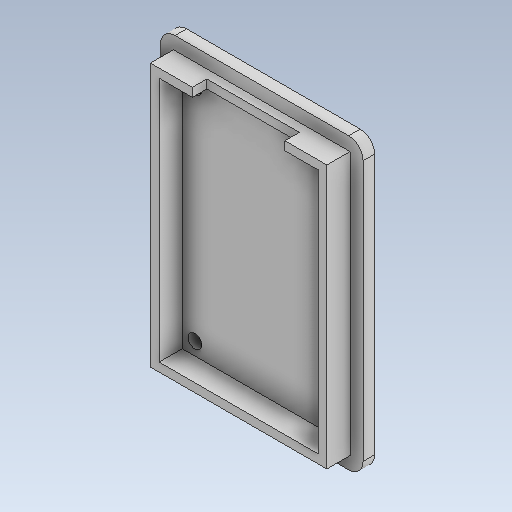
# Autodesk Inventor part: EnclosureTop
Saved by Autodesk Inventor 2020 (Build 240168000, 168)
## iProperties
Created: 2019-09-23
Part Number: EnclosureTop
Material: Generic
Document SubType Name: Modeling
Designer: veloxstatera
Density: 1 g/cm^3
Appearance: Default
Author: veloxstatera
Autodesk Inventor part; units mm, degrees
ref_plane "YZ Plane" through (0, 0, 0) normal (1, 0, 0) x (0, 1, 0)
ref_plane "XZ Plane" through (0, 0, 0) normal (0, 1, 0) x (-1, 0, 0)
ref_plane "XY Plane" through (0, 0, 0) normal (0, 0, 1) x (1, 0, 0)
sketch "Sketch1" plane through (0, 0, 0) normal (0, 0, 1) x (1, 0, 0)
  line L0 (-44.45, 63.5) -> (44.45, 63.5)
  line L1 (44.45, 63.5) -> (44.45, -63.5)
  line L2 (44.45, -63.5) -> (-44.45, -63.5)
  line L3 (-44.45, -63.5) -> (-44.45, 63.5)
  line L4 (0, 63.5) -> (0, -63.5) construction
  point P0 (0, 0)
  point P1 (0, 0)
  dimension "d0" = 88.9
  dimension "d1" = 127
  constraints: 10 end point, 3 midpoint, 2 parallel, 1 coincident, 1 horizontal, 1 perpendicular
  measures "d0" distance of L0.start L0.end
  measures "d1" distance of L0.end L1.end
extrude "Extrusion1" add sketch "Sketch1" along normal blind 5.08
fillet "Fillet1" radius 6.35 4 edges at (44.45, 63.5, 2.54) (-44.45, 63.5, 2.54) (44.45, -63.5, 2.54) (-44.45, -63.5, 2.54)
sketch "Sketch2" plane through (0, 0, 5.08) normal (0, 0, 1) x (1, 0, 0)
  line L0 (-38.735, 57.785) -> (38.735, 57.785)
  line L1 (38.735, 57.785) -> (38.735, -57.785)
  line L2 (38.735, -57.785) -> (-38.735, -57.785)
  line L3 (-38.735, -57.785) -> (-38.735, 57.785)
  line L4 (38.1, 63.5) -> (-38.1, 63.5) construction
  line L5 (44.45, -57.15) -> (44.45, 57.15) construction
  line L6 (0, 57.785) -> (0, -57.785) construction
  point P0 (0, 0)
  point P1 (0, 0)
  dimension "d5" = 77.47
  dimension "d6" = 115.57
  constraints: 10 end point, 3 midpoint, 2 parallel, 1 coincident, 1 horizontal, 1 perpendicular
  measures "d5" distance of L0.start L0.end
  measures "d6" distance of L0.end L1.end
extrude "Extrusion2" add sketch "Sketch2" along normal blind 10.16
sketch "Sketch3" plane through (0, 0, 15.24) normal (0, 0, 1) x (1, 0, 0)
  line L0 (-34.925, 53.975) -> (34.925, 53.975)
  line L1 (34.925, 53.975) -> (34.925, -53.975)
  line L2 (34.925, -53.975) -> (-34.925, -53.975)
  line L3 (-34.925, -53.975) -> (-34.925, 53.975)
  line L4 (0, -53.975) -> (0, 53.975) construction
  line L5 (38.735, 57.785) -> (-38.735, 57.785) projected
  line L6 (-38.735, 57.785) -> (-38.735, -57.785) projected
  point P0 (0, 0)
  point P1 (0, 0)
  dimension "d9" = 3.81
  dimension "d10" = 3.81
  constraints: 10 end point, 3 midpoint, 2 parallel, 1 coincident, 1 horizontal, 1 perpendicular
  measures "d9" distance between parallel lines of L5 L0
  measures "d10" distance between parallel lines of L6 L3
extrude "Extrusion3" cut sketch "Sketch3" against normal blind 10.16
sketch "Sketch4" plane through (-38.735, 57.785, 5.08) normal (0, 1, 0) x (1, 0, 0)
  line L0 (77.47, -10.16) -> (0, -10.16) projected
  line L1 (59.055, -10.16) -> (18.415, -10.16)
  line L2 (18.415, -10.16) -> (18.415, -3.81)
  line L3 (18.415, -3.81) -> (59.055, -3.81)
  line L4 (59.055, -3.81) -> (59.055, -10.16)
  point P0 (38.735, 5.08)
  point P1 (38.735, -10.16)
  dimension "d13" = 40.64
  dimension "d14" = 6.35
  constraints: 8 end point, 2 midpoint, 2 parallel, 1 horizontal, 1 perpendicular, 1 point on line
  measures "d13" distance of L2.end L3.end
  measures "d14" distance of L3.end L1.start
extrude "Extrusion4" cut sketch "Sketch4" against normal blind 10.16
sketch "Sketch5" plane through (0, 0, 5.08) normal (0, 0, 1) x (1, 0, 0)
  circle A0 centre (-29.325, 48.375) radius 3
  line L0 (20.32, 53.975) -> (-20.32, 53.975) construction
  line L1 (0, 53.975) -> (0, 7.6098) construction
  line L2 (0, 0) -> (12.3821, 0) construction
  line L3 (-34.925, 53.975) -> (-20.32, 53.975) construction
  line L4 (-34.925, -53.975) -> (-34.925, 53.975) construction
  circle A1 centre (29.325, 48.375) radius 3
  circle A2 centre (-29.325, -48.375) radius 3
  circle A3 centre (29.325, -48.375) radius 3
  dimension "d17" = 6
  dimension "d18" = 5.6
  dimension "d19" = 5.6
  constraints: 4 centre point, 4 end point, 3 symmetric about line, 1 horizontal, 1 midpoint, 1 vertical, 3 other
  measures "d17" diameter of A0
  measures "d18" distance from line of L3 A0.centre
  measures "d19" distance from line of L4 A0.centre
extrude "Extrusion5" cut sketch "Sketch5" against normal blind 10
body "Solid1"
